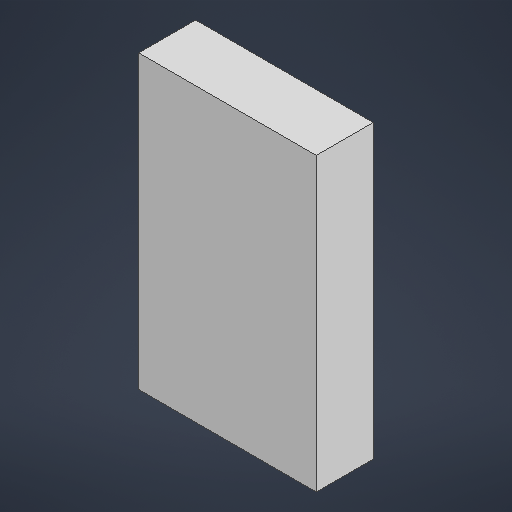
# Autodesk Inventor part: SAFRS-P-0026
Saved by Autodesk Inventor 2026.2 (Build 302298000, 298)
## iProperties
Created: 2025-11-26
Part Number: SAFRS-P-0026
Material: 일반
Document SubType Name: Modeling
Designer: jaewook
Density: 1 g/cm^3
Appearance: 기본값
Author: jaewook
Title: Battery Pack 2
Autodesk Inventor part; units mm, degrees
ref_plane "YZ Plane" through (0, 0, 0) normal (1, 0, 0) x (0, 1, 0)
ref_plane "XZ Plane" through (0, 0, 0) normal (0, 1, 0) x (-1, 0, 0)
ref_plane "XY Plane" through (0, 0, 0) normal (0, 0, 1) x (1, 0, 0)
sketch "스케치1" plane through (0, 0, 0) normal (0, 0, 1) x (1, 0, 0)
  line L0 (33.5, -55) -> (-33.5, -55)
  line L1 (-33.5, -55) -> (-33.5, 55)
  line L2 (-33.5, 55) -> (33.5, 55)
  line L3 (33.5, 55) -> (33.5, -55)
  line L4 (33.5, -55) -> (-33.5, 55) construction
  line L5 (-33.5, -55) -> (33.5, 55) construction
  point P0 (0, 0)
  dimension "d0" = 67
  dimension "d1" = 110
  constraints: 12 end point, 2 midpoint, 2 parallel, 1 horizontal, 1 perpendicular
  measures "d0" distance of L1.end L2.end
  measures "d1" distance of L0.end L1.end
extrude "돌출1" add sketch "스케치1" along normal blind 21.5
